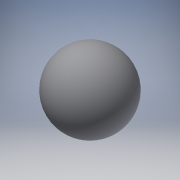
# Autodesk Inventor part: Boule
Saved by Autodesk Inventor 2017 (Build 210142000, 142)
## iProperties
Part Number: Boule
Material: Générique
Document SubType Name: Modeling
Designer: Thomas
Density: 1 g/cm^3
Appearance: Par défaut
Author: Thomas
Autodesk Inventor part; units mm, degrees
ref_plane "YZ Plane" through (0, 0, 0) normal (1, 0, 0) x (0, 1, 0)
ref_plane "XZ Plane" through (0, 0, 0) normal (0, 1, 0) x (-1, 0, 0)
ref_plane "XY Plane" through (0, 0, 0) normal (0, 0, 1) x (1, 0, 0)
sketch "Esquisse1" plane through (0, 0, 0) normal (0, 1, 0) x (-1, 0, 0)
  arc A0 (-22.5, 0) -> (22.5, 0) centre (0, 0) ccw
  line L0 (22.5, 0) -> (-22.5, 0) construction
  line L1 (22.5, 0) -> (-22.5, 0)
  dimension "d0" = 45
  constraints: 4 end point, 2 point on circle, 1 centre point, 1 coincident, 1 collinear
  measures "d0" diameter of A0
revolve "Révolution1" add sketch "Esquisse1" angle 360 about axis through (-22.5, 0, 0) along (1, 0, 0)
